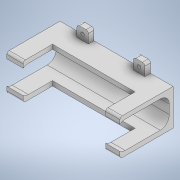
# Autodesk Inventor part: Porta pilas
Saved by Autodesk Inventor 2020 (Build 240168000, 168)
## iProperties
Created: 2020-11-22
Part Number: Porta pilas
Material: Generic
Document SubType Name: Modeling
Designer: michelin
Density: 1 g/cm^3
Appearance: Default
Author: michelin
Autodesk Inventor part; units mm, degrees
ref_plane "YZ Plane" through (0, 0, 0) normal (1, 0, 0) x (0, 1, 0)
sketch "Sketch1" plane through (0, 0, 0) normal (0, 0, 1) x (1, 0, 0)
  line L0 (29.367, 37.7153) -> (29.0801, 37.3058)
  arc A0 (25.6709, 43.8574) -> (29.0801, 37.3058) centre (33.6709, 43.8574) ccw
  line L1 (25.6709, 51.8574) -> (25.6709, 43.8574)
  line L2 (25.6709, 43.8574) -> (25.6709, 51.8574)
  arc A1 (33.6709, 59.8574) -> (25.6709, 51.8574) centre (33.6709, 51.8574) ccw
  line L3 (33.6709, 59.8574) -> (64.6709, 59.8574)
  arc A2 (72.6709, 51.8574) -> (64.6709, 59.8574) centre (64.6709, 51.8574) ccw
  line L4 (72.6709, 43.8574) -> (72.6709, 51.8574)
  line L5 (72.6709, 51.8576) -> (72.6709, 43.8574)
  arc A3 (64.6709, 35.8574) -> (72.6709, 43.8574) centre (64.6709, 43.8574) ccw
  arc A4 (33.6709, 59.8574) -> (25.6709, 51.8574) centre (33.6709, 51.8574) ccw
  arc A5 (25.6709, 43.8574) -> (33.6709, 35.8574) centre (33.6709, 43.8574) ccw
  arc A6 (64.6709, 35.8574) -> (72.6709, 43.8574) centre (64.6709, 43.8574) ccw
  arc A7 (72.6709, 51.8574) -> (64.6709, 59.8574) centre (64.6709, 51.8574) ccw
  line L6 (33.6709, 35.8574) -> (64.6709, 35.8574)
  line L7 (33.6709, 35.8574) -> (50.3633, 35.8574)
  line L8 (50.3633, 59.8574) -> (50.3633, 35.8574)
  line L9 (25.6709, 47.8574) -> (50.3633, 47.8574)
  line L10 (84.9941, 47.8575) -> (84.9941, 63.8575)
  line L11 (84.9941, 63.8575) -> (184.9941, 63.8575)
  line L12 (84.9941, 47.8575) -> (84.9941, 31.8575)
  line L13 (84.9941, 31.8575) -> (184.9941, 31.8575)
  line L14 (184.9941, 31.8575) -> (184.9941, 63.8575)
  line L15 (184.9941, 31.8575) -> (164.9941, 31.8575)
  line L16 (164.9941, 31.8575) -> (164.9941, 21.8575)
  line L17 (164.9941, 21.8575) -> (154.9941, 21.8575)
  line L18 (154.9941, 21.8575) -> (154.9941, 31.8575)
  line L19 (84.9941, 31.8575) -> (104.9941, 31.8575)
  line L20 (104.9941, 31.8575) -> (104.9941, 21.8575)
  line L21 (104.9941, 21.8575) -> (114.9941, 21.8575)
  line L22 (114.9941, 21.8575) -> (114.9941, 31.8575)
  line L23 (184.9941, 63.8575) -> (164.9941, 63.8575)
  line L24 (164.9941, 63.8575) -> (164.9941, 73.8575)
  line L25 (164.9941, 73.8575) -> (154.9941, 73.8575)
  line L26 (154.9941, 73.8575) -> (154.9941, 63.8575)
  line L27 (84.9941, 63.8575) -> (104.9941, 63.8575)
  line L28 (104.9941, 63.8575) -> (104.9941, 73.8575)
  line L29 (104.9941, 73.8575) -> (114.9941, 73.8575)
  line L30 (114.9941, 73.8575) -> (114.9941, 63.8575)
  line L31 (104.9941, 63.8575) -> (109.9941, 63.8575)
  line L32 (104.9941, 31.8575) -> (109.9941, 31.8575)
  line L33 (104.9941, 31.8575) -> (109.9941, 31.8575)
  line L34 (109.9941, 26.8575) -> (109.9941, 31.8575)
  line L35 (154.9941, 63.8575) -> (159.9941, 63.8575)
  line L36 (154.9941, 31.8575) -> (159.9941, 31.8575)
  circle A8 centre (109.9941, 68.8575) radius 1.5875
  circle A9 centre (159.9941, 68.8575) radius 1.5875
  circle A10 centre (109.9941, 26.8575) radius 1.5875
  circle A11 centre (159.9941, 26.8575) radius 1.5875
  point P0 (0, 0)
  constraints: 74 end point, 22 point on line, 18 point on circle, 12 centre point, 10 perpendicular, 5 coincident, 3 horizontal, 2 collinear, 2 midpoint, 1 concentric, 1 vertical
sketch "Sketch2" plane through (0, 0, 0) normal (0, 0, 1) x (1, 0, 0)
  line L0 (29.367, 37.7153) -> (29.0801, 37.3058)
  arc A0 (25.6709, 43.8574) -> (29.0801, 37.3058) centre (33.6709, 43.8574) ccw
  line L1 (25.6709, 51.8574) -> (25.6709, 43.8574)
  line L2 (25.6709, 43.8574) -> (25.6709, 51.8574)
  arc A1 (33.6709, 59.8574) -> (25.6709, 51.8574) centre (33.6709, 51.8574) ccw
  line L3 (33.6709, 59.8574) -> (64.6709, 59.8574)
  arc A2 (72.6709, 51.8574) -> (64.6709, 59.8574) centre (64.6709, 51.8574) ccw
  line L4 (72.6709, 43.8574) -> (72.6709, 51.8574)
  line L5 (72.6709, 51.8576) -> (72.6709, 43.8574)
  arc A3 (64.6709, 35.8574) -> (72.6709, 43.8574) centre (64.6709, 43.8574) ccw
  arc A4 (33.6709, 59.8574) -> (25.6709, 51.8574) centre (33.6709, 51.8574) ccw
  arc A5 (25.6709, 43.8574) -> (33.6709, 35.8574) centre (33.6709, 43.8574) ccw
  arc A6 (64.6709, 35.8574) -> (72.6709, 43.8574) centre (64.6709, 43.8574) ccw
  arc A7 (72.6709, 51.8574) -> (64.6709, 59.8574) centre (64.6709, 51.8574) ccw
  line L6 (33.6709, 35.8574) -> (64.6709, 35.8574)
  line L7 (33.6709, 35.8574) -> (50.3633, 35.8574)
  line L8 (50.3633, 59.8574) -> (50.3633, 35.8574)
  line L9 (25.6709, 47.8574) -> (50.3633, 47.8574)
  line L10 (84.9941, 47.8575) -> (84.9941, 63.8575)
  line L11 (84.9941, 63.8575) -> (184.9941, 63.8575)
  line L12 (84.9941, 47.8575) -> (84.9941, 31.8575)
  line L13 (84.9941, 31.8575) -> (184.9941, 31.8575)
  line L14 (184.9941, 31.8575) -> (184.9941, 63.8575)
  line L15 (184.9941, 31.8575) -> (164.9941, 31.8575)
  line L16 (164.9941, 31.8575) -> (164.9941, 21.8575)
  line L17 (164.9941, 21.8575) -> (154.9941, 21.8575)
  line L18 (154.9941, 21.8575) -> (154.9941, 31.8575)
  line L19 (84.9941, 31.8575) -> (104.9941, 31.8575)
  line L20 (104.9941, 31.8575) -> (104.9941, 21.8575)
  line L21 (104.9941, 21.8575) -> (114.9941, 21.8575)
  line L22 (114.9941, 21.8575) -> (114.9941, 31.8575)
  line L23 (184.9941, 63.8575) -> (164.9941, 63.8575)
  line L24 (164.9941, 63.8575) -> (164.9941, 73.8575)
  line L25 (164.9941, 73.8575) -> (154.9941, 73.8575)
  line L26 (154.9941, 73.8575) -> (154.9941, 63.8575)
  line L27 (84.9941, 63.8575) -> (104.9941, 63.8575)
  line L28 (104.9941, 63.8575) -> (104.9941, 73.8575)
  line L29 (104.9941, 73.8575) -> (114.9941, 73.8575)
  line L30 (114.9941, 73.8575) -> (114.9941, 63.8575)
  line L31 (104.9941, 63.8575) -> (109.9941, 63.8575)
  line L32 (104.9941, 31.8575) -> (109.9941, 31.8575)
  line L33 (104.9941, 31.8575) -> (109.9941, 31.8575)
  line L34 (109.9941, 26.8575) -> (109.9941, 31.8575)
  line L35 (154.9941, 63.8575) -> (159.9941, 63.8575)
  line L36 (154.9941, 31.8575) -> (159.9941, 31.8575)
  circle A8 centre (109.9941, 68.8575) radius 1.5875
  circle A9 centre (159.9941, 68.8575) radius 1.5875
  circle A10 centre (109.9941, 26.8575) radius 1.5875
  circle A11 centre (159.9941, 26.8575) radius 1.5875
  point P0 (0, 0)
  constraints: 74 end point, 22 point on line, 18 point on circle, 12 centre point, 10 perpendicular, 5 coincident, 3 horizontal, 2 collinear, 2 midpoint, 1 concentric, 1 vertical
extrude "Extrusion1" add sketch "Sketch1" along normal blind 47 contours L10 L11 L14 L13 L12
extrude "Extrusion2" add sketch "Sketch2" along normal blind 5 contours L28 L29 L30 L11 | L13 L22 L21 L20 | L26 L25 L24 L11 | L13 L16 L17 L18
ref_plane "Work Plane1" through (84.9941, 63.8575, 47) normal (0, 1, 0) x (1, 0, 0)
sketch "Sketch3" plane through (84.9941, 63.8575, 47) normal (0, 1, 0) x (1, 0, 0)
  point P0 (-84.9941, 47)
ref_plane "Work Plane2" through (84.9941, 31.8575, 0) normal (-1, 0, 0) x (0, 0, 1)
sketch "Sketch4" plane through (84.9941, 31.8575, 0) normal (-1, 0, 0) x (0, 0, 1)
  line L0 (7.0327, 5.966) -> (6.7458, 5.5565)
  arc A0 (3.3366, 12.1082) -> (6.7458, 5.5565) centre (11.3366, 12.1082) ccw
  line L1 (3.3366, 20.1082) -> (3.3366, 12.1082)
  line L2 (3.3366, 12.1082) -> (3.3366, 20.1082)
  arc A1 (11.3366, 28.1082) -> (3.3366, 20.1082) centre (11.3366, 20.1082) ccw
  line L3 (11.3366, 28.1082) -> (42.3366, 28.1082)
  arc A2 (50.3366, 20.1082) -> (42.3366, 28.1082) centre (42.3366, 20.1082) ccw
  line L4 (50.3366, 12.1082) -> (50.3366, 20.1082)
  line L5 (50.3366, 20.1083) -> (50.3366, 12.1082)
  arc A3 (42.3366, 4.1082) -> (50.3366, 12.1082) centre (42.3366, 12.1082) ccw
  arc A4 (11.3366, 28.1082) -> (3.3366, 20.1082) centre (11.3366, 20.1082) ccw
  arc A5 (3.3366, 12.1082) -> (11.3366, 4.1082) centre (11.3366, 12.1082) ccw
  arc A6 (42.3366, 4.1082) -> (50.3366, 12.1082) centre (42.3366, 12.1082) ccw
  arc A7 (50.3366, 20.1082) -> (42.3366, 28.1082) centre (42.3366, 20.1082) ccw
  line L6 (11.3366, 4.1082) -> (42.3366, 4.1082)
  line L7 (11.3366, 4.1082) -> (28.029, 4.1082)
  line L8 (28.029, 28.1082) -> (28.029, 4.1082)
  line L9 (3.3366, 16.1082) -> (28.029, 16.1082)
  point P0 (0, -31.8575)
  point P1 (50.3366, 20.1082)
  constraints: 20 end point, 18 point on circle, 8 centre point, 6 point on line, 4 coincident, 2 collinear, 2 midpoint, 1 concentric, 1 horizontal, 1 perpendicular
extrude "Extrusion3" cut sketch "Sketch4" against normal blind 110
sketch "Sketch5" plane through (84.9941, 63.8575, 47) normal (0, 1, 0) x (1, 0, 0)
  line L0 (14.3535, -16.4072) -> (87.4033, -16.4072)
  line L1 (87.4033, -16.4072) -> (87.4033, 25.9617)
  line L2 (87.4033, 25.9617) -> (14.3535, 25.9617)
  line L3 (14.3535, 25.9617) -> (14.3535, -16.4072)
  point P0 (-84.9941, 47)
  constraints: 8 end point, 2 parallel, 1 horizontal, 1 perpendicular
extrude "Extrusion4" cut sketch "Sketch5" against normal blind 40
fillet "Fillet1" radius 2 4 edges at (92.1709, 63.8575, 47) (178.6957, 63.8575, 47) (178.6957, 31.8575, 47) (92.1709, 31.8575, 47)
fillet "Fillet2" radius 2 8 edges at (164.9941, 73.8575, 2.5) (154.9941, 73.8575, 2.5) (114.9941, 73.8575, 2.5) (104.9941, 73.8575, 2.5) (164.9941, 21.8575, 2.5) (154.9941, 21.8575, 2.5) (114.9941, 21.8575, 2.5) (104.9941, 21.8575, 2.5)
body "Solid1"
